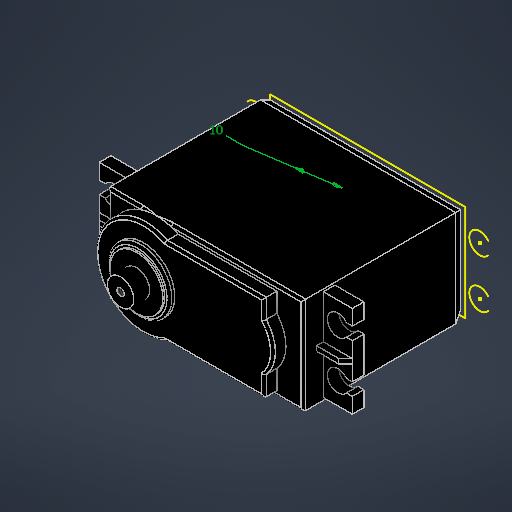
# Autodesk Inventor part: Servo Skiba
Saved by Autodesk Inventor 2027.1 (Build 311270010, 270A)
## iProperties
Created: 2020-09-10
Part Number: Servo Skiba
Material: Generic
Document SubType Name: Modeling
Designer: 239tr
Density: 1 g/cm^3
Appearance: Anodized - Black
Mass: 29.5422 g
Surface Area: 66.2548 cm^2
Volume: 29.5422 cm^3
Author: 239tr
Autodesk Inventor part; units mm, degrees
ref_plane "YZ Plane" through (0, 0, 0) normal (1, 0, 0) x (0, 1, 0)
sketch "Sketch1" plane through (0, 0, 0) normal (0, 0, 1) x (1, 0, 0)
  line L0 (0, 0) -> (40.5, 0)
  line L1 (40.5, 0) -> (40.5, 20)
  line L2 (40.5, 20) -> (0, 20)
  line L3 (0, 20) -> (0, 0)
  dimension "d0" = 40.5
  dimension "d1" = 20
  constraints: 8 end point, 2 parallel, 1 horizontal, 1 perpendicular
  measures "d0" distance of L2.end L1.end
  measures "d1" distance of L1.end L0.end
extrude "Extrusion1" add sketch "Sketch1" along normal blind 33.6
chamfer "Chamfer1" distance 1 angle 63.4 3 edges at (20.25, 20, 0) (40.5, 10, 0) (20.25, 0, 0) measured on face at (40, 10, 0) measured on face at (20.25, 0.5, 0) measured on face at (20.25, 19.5, 0)
sketch "Sketch2" plane through (0, 0, 33.6) normal (-1, 0, 0) x (0, 0, 1)
  line L0 (-33.6, 19) -> (-33.6, 1)
  line L1 (-33.6, 6.65) -> (-29.6, 6.65)
  line L2 (-29.6, 6.65) -> (-29.6, 13.35)
  line L3 (-29.6, 13.35) -> (-33.6, 13.35)
  line L4 (-33.6, 13.35) -> (-33.6, 6.65)
  line L5 (-31.603046, 0) -> (0, 0)
  point P0 (-33.6, 0)
  point P1 (-33.6, 13.35)
  dimension "d7" = 4
  dimension "d8" = 6.7
  dimension "d9" = 6.65
  constraints: 8 end point, 2 parallel, 1 horizontal, 1 perpendicular, 1 point on line
  measures "d7" distance of L3.end L2.end
  measures "d8" distance of L2.end L1.end
  measures "d9" distance between parallel lines of L5 L1
extrude "Extrusion2" add sketch "Sketch2" along normal blind 1.6
ref_plane "Work Plane2" through (-1.6, 13.35, 2) normal (-1, 0, 0) x (0, 0, 1)
sketch "Sketch5" plane through (-1.6, 13.35, 2) normal (-1, 0, 0) x (0, 0, 1)
  line L0 (2, 0) -> (2, -6.7) projected
  line L1 (2, 0) -> (-2, 0) projected
  line L2 (2, -6.7) -> (-2, -6.7)
  line L3 (-2, -6.7) -> (-2, 0)
  line L4 (-2, 0) -> (2, 0)
  line L5 (2, 0) -> (2, -6.7)
  point P0 (-2, -13.35)
  constraints: 8 end point, 2 parallel, 1 horizontal, 1 perpendicular
ref_plane "Work Plane3" through (-6, 13.35, 2) normal (-1, 0, 0) x (0, 0, 1)
sketch "Sketch6" plane through (-6, 13.35, 2) normal (-1, 0, 0) x (0, 0, 1)
  line L0 (-2, -6.7) -> (-2, 0) construction
  line L1 (-2, -6.7) -> (2, -6.7) construction
  line L2 (2, 0) -> (2, -6.7) construction
  line L3 (2, 0) -> (-2, 0) construction
  line L4 (1, -6) -> (-1.5, -6)
  line L5 (-1.5, -6) -> (-1.5, -0.7)
  line L6 (-1.5, -0.7) -> (1, -0.7)
  line L7 (1, -0.7) -> (1, -6)
  point P0 (-2, -13.35)
  dimension "d18" = 2.5
  dimension "d19" = 5.3
  dimension "d20" = 0.7
  dimension "d27" = 0.5
  constraints: 8 end point, 2 parallel, 1 horizontal, 1 perpendicular
  measures "d18" distance of L5.end L6.end
  measures "d19" distance of L4.end L5.end
  measures "d20" distance between parallel lines of L1 L4
  measures "d27" distance between parallel lines of L0 L5
loft "Loft1" add profiles "Sketch5", "Sketch6" separate body
ref_plane "Work Plane4" through (0, 0, 27.05) normal (0, 0, -1) x (-1, 0, 0)
sketch "Sketch7" plane through (0, 0, 27.05) normal (0, 0, -1) x (-1, 0, 0)
  line L0 (-40.5, 0) -> (-40.5, 20) construction
  line L1 (-40.5, 20) -> (0, 20) construction
  line L2 (0, 20) -> (0, 0) construction
  line L3 (0, 0) -> (-40.5, 0) construction
  line L4 (0, 0.5) -> (6, 0.5)
  line L5 (6, 0.5) -> (6, 19.5)
  line L6 (6, 19.5) -> (0, 19.5)
  line L7 (0, 19.5) -> (0, 0.5)
  arc A0 (4.749971, 16.3) -> (4.749971, 13.7) centre (3, 15) ccw
  arc A1 (4.749971, 6.3) -> (4.749971, 3.7) centre (3, 5) ccw
  line L8 (-40.5, 0.5) -> (-46.5, 0.5)
  line L9 (-46.5, 0.5) -> (-46.5, 19.5)
  line L10 (-46.5, 19.5) -> (-40.5, 19.5)
  line L11 (-40.5, 19.5) -> (-40.5, 0.5)
  arc A2 (-45.249971, 13.7) -> (-45.249971, 16.3) centre (-43.5, 15) ccw
  arc A3 (-45.249971, 3.7) -> (-45.249971, 6.3) centre (-43.5, 5) ccw
  line L12 (6, 16.3) -> (4.749971, 16.3)
  line L13 (6, 13.7) -> (4.749971, 13.7)
  line L14 (6, 6.3) -> (4.749971, 6.3)
  line L15 (6, 3.7) -> (4.749971, 3.7)
  line L16 (-46.5, 3.7) -> (-45.249971, 3.7)
  line L17 (-46.5, 6.3) -> (-45.249971, 6.3)
  line L18 (-46.5, 13.7) -> (-45.249971, 13.7)
  line L19 (-46.5, 16.3) -> (-45.249971, 16.3)
  dimension "d28" = 6
  dimension "d29" = 19
  dimension "d30" = 0.5
  dimension "d31" = 4.36
  dimension "d32" = 4.36
  dimension "d33" = 4.5
  dimension "d34" = 3
  dimension "d35" = 4.5
  dimension "d36" = 3
  dimension "d37" = 6
  dimension "d38" = 19
  dimension "d39" = 0.5
  dimension "d40" = 4.36
  dimension "d41" = 4.36
  dimension "d42" = 4.5
  dimension "d43" = 3
  dimension "d44" = 3
  dimension "d45" = 4.5
  dimension "d47" = 3.7
  dimension "d48" = 6.3
  dimension "d49" = 13.7
  dimension "d50" = 16.3
  dimension "d51" = 3.7
  dimension "d52" = 6.3
  dimension "d53" = 13.7
  dimension "d54" = 16.3
  constraints: 32 end point, 10 parallel, 10 point on line, 8 point on circle, 4 centre point, 4 perpendicular, 2 horizontal
  measures "d28" distance of L6.end L5.end
  measures "d29" distance of L5.end L4.end
  measures "d30" distance from line of point (0, 0) L4
  measures "d31" diameter of A0
  measures "d32" diameter of A1
  measures "d33" distance from line of L6 A0.centre
  measures "d34" distance from line of A0.centre L5
  measures "d35" distance from line of L4 A1.centre
  measures "d36" distance from line of L5 A1.centre
  measures "d37" distance of L9.end L10.end
  measures "d38" distance of L8.end L9.end
  measures "d39" distance from line of L0.start L8
  measures "d40" diameter of A2
  measures "d41" diameter of A3
  measures "d42" distance from line of L10 A2.centre
  measures "d43" distance from line of L9 A2.centre
  measures "d44" distance from line of L9 A3.centre
  measures "d45" distance from line of L8 A3.centre
  measures "d47" distance from line of L15 point (0, 0)
  measures "d48" distance from line of L14 point (0, 0)
  measures "d49" distance from line of L13 point (0, 0)
  measures "d50" distance from line of L12 point (0, 0)
  measures "d51" distance from line of L16 L0.start
  measures "d52" distance from line of L17 L0.start
  measures "d53" distance from line of L18 L0.start
  measures "d54" distance from line of L19 L0.start
extrude "Extrusion3" add sketch "Sketch7" against normal blind 2.4 contours L7 L6 L5 L12 A0 L13 L14 A1 L15 L4 | L8 L9 L16 A3 L17 L18 A2 L19 L10 L11 bodies 1
sketch "Sketch8" plane through (0, 0, 29.45) normal (0, 0, 1) x (1, 0, 0)
  line L0 (-6, 12.65) -> (-6, 7.35) projected
  line L1 (0, 19.5) -> (0, 0.5) projected
  line L2 (-6, 9.5) -> (0, 9.5)
  line L3 (0, 9.5) -> (0, 10.5)
  line L4 (0, 10.5) -> (-6, 10.5)
  line L5 (-6, 10.5) -> (-6, 9.5)
  line L6 (40.5, 19.5) -> (40.5, 0.5) projected
  line L7 (46.5, 6.3) -> (46.5, 13.7) projected
  line L8 (40.5, 9.5) -> (46.5, 9.5)
  line L9 (46.5, 9.5) -> (46.5, 10.5)
  line L10 (46.5, 10.5) -> (40.5, 10.5)
  line L11 (40.5, 10.5) -> (40.5, 9.5)
  point P0 (0, 0)
  point P1 (40.5, 0)
  point P2 (0, 9.5)
  dimension "d57" = 1
  dimension "d58" = 1
  dimension "d59" = 9.5
  dimension "d60" = 9.5
  constraints: 16 end point, 4 parallel, 4 point on line, 2 horizontal, 2 perpendicular
  measures "d57" distance of L3.end L2.end
  measures "d58" distance between parallel lines of L8 L10
  measures "d59" distance from line of L2 point (0, 0)
  measures "d60" distance from line of L8 point (40.5, 0)
extrude "Extrusion4" add sketch "Sketch8" along normal blind 1.4 bodies 1
chamfer "Chamfer2" distance 1.5 distance2 1.4 1 edges at (-6, 10, 30.85) measured on face at (-5.5, 10, 30.85)
chamfer "Chamfer3" distance 1.5 distance2 1.4 1 edges at (46.5, 10, 30.85) measured on face at (46, 10, 30.85)
sketch "Sketch9" plane through (0, 0, 33.6) normal (0, 0, 1) x (1, 0, 0)
  arc A0 (14.500567, 18.93) -> (14.500567, 1.07) centre (10, 10) ccw
  line L0 (40.5, 20) -> (0, 20)
  line L1 (0, 0) -> (40.5, 0)
  line L2 (0, 20) -> (0, 0)
  arc A1 (35, 5.071552) -> (35, 14.928448) centre (29.48, 10) ccw
  line L3 (35, 14.928448) -> (35, 5.071552) construction
  line L4 (35, 14.928448) -> (44.856896, 14.928448) construction
  line L5 (14.500567, 18.93) -> (35, 18.93)
  line L6 (35, 18.93) -> (35, 14.928448)
  line L7 (14.500567, 1.07) -> (35, 1.07)
  line L8 (35, 1.07) -> (35, 5.071552)
  dimension "d69" = 90
  dimension "d70" = 7.4
  dimension "d71" = 1.07
  dimension "d72" = 1.07
  dimension "d73" = 35
  dimension "d74" = 29.48
  dimension "d75" = 10
  constraints: 12 end point, 4 point on circle, 3 horizontal, 3 perpendicular, 3 tangent, 2 centre point
  measures "d69" angle of L3 L4
  measures "d70" radius of A1
  measures "d71" distance between parallel lines of L1 L7
  measures "d72" distance between parallel lines of L0 L5
  measures "d73" distance between parallel lines of L6 L2
  measures "d74" distance from line of L2 A1.centre
  measures "d75" distance from line of L0 A1.centre
extrude "Extrusion5" add sketch "Sketch9" along normal blind 2.68 contours L5 L6 A1 L8 L7 A0 bodies 1
sketch "Sketch10" plane through (0, 0, 36.28) normal (0, 0, 1) x (1, 0, 0)
  circle A0 centre (10, 10) radius 6.5
  arc A1 (14.500567, 18.93) -> (14.500567, 1.07) centre (10, 10) ccw
  point P0 (0, 0)
  dimension "d78" = 13
  constraints: 1 centre point, 1 concentric
  measures "d78" diameter of A0
extrude "Extrusion6" add sketch "Sketch10" along normal blind 1.1 bodies 1
sketch "Sketch11" plane through (10, 10, 37.38) normal (0, 0, 1) x (1, 0, 0)
  circle A0 centre (0, 0) radius 5.5
  circle A1 centre (0, 0) radius 6.5 projected
  point P0 (-10, -10)
  dimension "d81" = 11
  constraints: 1 centre point, 1 concentric
  measures "d81" diameter of A0
extrude "Extrusion7" add sketch "Sketch11" along normal blind 0.35 contours A0 bodies 1
sketch "Sketch12" plane through (10, 10, 37.73) normal (0, 0, 1) x (1, 0, 0)
  circle A0 centre (0, 0) radius 2.75
  circle A1 centre (0, 0) radius 5.5 projected
  point P0 (-10, -10)
  dimension "d84" = 5.5
  constraints: 1 centre point, 1 concentric
  measures "d84" diameter of A0
extrude "Extrusion8" add sketch "Sketch12" along normal blind 3.3 contours A0 bodies 1
sketch "Sketch13" plane through (10, 10, 41.03) normal (0, 0, 1) x (1, 0, 0)
  point P0 (-10, -10)
  point P1 (0, 0)
  point P2 (0, 0)
  constraints: 1 coincident
hole "Hole1" at (10, 10, 41.03) direction (0, 0, -1) diameter 1.567 depth 6 tip angle 118 bodies 1 thread size "M2x0.4" class "6H" standard "ANSI Metric M Profile"
fillet "Fillet1" radius 0.5 14 edges at (3.5, 10, 37.38) (0, 10, 36.28) (24.7503, 1.07, 36.28) (35, 3.0708, 36.28) (36.88, 10, 36.28) (35, 16.9292, 36.28) (24.7503, 18.93, 36.28) (25.25, 0, 33.6) (5, 0, 33.6) (0, 5, 33.6) (0, 15, 33.6) (5, 20, 33.6) (25.25, 20, 33.6) (40.5, 10, 33.6)
sketch "Sketch14" plane through (0, 0, 0) normal (0, 0, -1) x (-1, 0, 0)
  line L0 (0, 19) -> (0, 20)
  line L1 (0, 19) -> (0, 13.35)
  line L2 (0, 13.35) -> (0, 6.65)
  line L3 (0, 6.65) -> (0, 1)
  line L4 (0, 0) -> (0, 1)
  line L5 (-40.5, 0) -> (0, 0)
  line L6 (-40.5, 20) -> (-40.5, 0)
  line L7 (0, 20) -> (-40.5, 20)
  circle A0 centre (-10, 10) radius 2.75
  arc A1 (4.749971, 6.3) -> (4.749971, 3.7) centre (3, 5) ccw
  arc A2 (4.749971, 16.3) -> (4.749971, 13.7) centre (3, 15) ccw
  arc A3 (-45.249971, 3.7) -> (-45.249971, 6.3) centre (-43.5, 5) ccw
  arc A4 (-45.249971, 13.7) -> (-45.249971, 16.3) centre (-43.5, 15) ccw
  circle A5 centre (-10, 10) radius 5
  line L8 (6, 10.5) -> (0, 10.5)
  line L9 (6, 10.5) -> (6, 9.5)
  line L10 (0, 9.5) -> (6, 9.5)
  line L11 (0, 10.5) -> (0, 9.5)
  dimension "d95" = 10
  constraints: 1 centre point, 1 coincident
  measures "d95" diameter of A5
equation "\"d32\" = d31"
equation "\"d35\" = d33"
equation "\"d38\" = d29"
equation "\"d40\" = d31"
equation "\"d41\" = d31"
equation "\"d42\" = d33"
equation "\"d45\" = d33"
equation "\"d51\" = d47"
equation "\"d52\" = d48"
equation "\"d53\" = d49"
equation "\"d54\" = d50"
equation "\"d60\" = d59"
equation "\"d72\" = d71"
body "Solid1"
body "Solid2"
